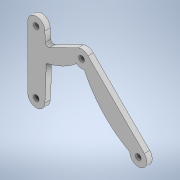
# Autodesk Inventor part: Bracket Concept MK5
Saved by Autodesk Inventor 2021 (Build 250183000, 183)
## iProperties
Created: 2021-05-11
Part Number: Bracket Concept MK5
Material: Generic
Document SubType Name: Modeling
Designer: Jawal
Density: 1 g/cm^3
Appearance: Default
Author: Jawal
Autodesk Inventor part; units mm, degrees
ref_plane "YZ Plane" through (0, 0, 0) normal (1, 0, 0) x (0, 1, 0)
ref_plane "XZ Plane" through (0, 0, 0) normal (0, 1, 0) x (-1, 0, 0)
ref_plane "XY Plane" through (0, 0, 0) normal (0, 0, 1) x (1, 0, 0)
sketch "Sketch1" plane through (0, 0, 0) normal (0, 0, 1) x (1, 0, 0)
  line L0 (-110, 70) -> (110, 70) construction
  line L1 (110, 70) -> (110, -70) construction
  line L2 (110, -70) -> (-110, -70) construction
  line L3 (-110, -70) -> (-110, 70) construction
  circle A0 centre (-90, 55) radius 5
  circle A1 centre (-90, -55) radius 5
  circle A2 centre (90, -55) radius 5
  circle A3 centre (-10, 45) radius 5
  line L4 (-67, 0) -> (-42, 0) construction
  line L5 (-42, 0) -> (-42, -30) construction
  line L6 (-42, -30) -> (-67, -30) construction
  line L7 (-67, -30) -> (-67, 0) construction
  circle A4 centre (-54.5, -11) radius 10 construction
  circle A5 centre (-63.5044, -24.4163) radius 3 construction
  circle A6 centre (-57.3559, -26.4695) radius 3 construction
  circle A7 centre (-51.263, -24.6531) radius 3 construction
  circle A8 centre (-45.3418, -26.5938) radius 3 construction
  arc A9 (-75, 55) -> (-105, 55) centre (-90, 55) ccw
  arc A10 (-105, -55) -> (-75, -55) centre (-90, -55) ccw
  arc A11 (75, -55) -> (100.6048, -44.3916) centre (90, -55) ccw
  line L8 (-105, 55) -> (-105, -55)
  line L9 (-66.6851, 34.062) -> (-16.5712, 58.484)
  arc A12 (-69.8902, 7.8152) -> (-19.1143, 33.0484) centre (-96.0046, 124.0681) ccw
  arc A13 (-75, -55) -> (-72.8183, 4.1339) centre (-763.2438, 0) ccw
  arc A14 (-73.8678, 38.2795) -> (-75, 55) centre (-763.2438, 0) ccw
  line L10 (1.1803, 55) -> (100.6048, -44.3916)
  arc A15 (-5.3208, 30.7166) -> (75, -55) centre (163.06, 108.0073) ccw
  arc A16 (-19.1143, 33.0484) -> (-5.3208, 30.7166) centre (-10, 45) ccw
  arc A17 (1.1803, 55) -> (-16.5712, 58.484) centre (-10, 45) ccw
  arc A18 (-73.8678, 38.2795) -> (-66.6851, 34.062) centre (-68.8755, 38.5567) ccw
  arc A19 (-69.8902, 7.8152) -> (-72.8183, 4.1339) centre (-69.0683, 4.1564) ccw
  point P0 (0, 0)
  dimension "d1" = 70
  dimension "d2" = 70
  dimension "d3" = 110
  dimension "d4" = 110
  dimension "d5" = 10
  dimension "d6" = 10
  dimension "d7" = 10
  dimension "d8" = 10
  dimension "d9" = 55
  dimension "d10" = 55
  dimension "d11" = 55
  dimension "d12" = 180
  dimension "d13" = 90
  dimension "d14" = 90
  dimension "d15" = 10
  dimension "d16" = 45
  dimension "d17" = 42
  dimension "d18" = 30
  dimension "d19" = 0
  dimension "d20" = 25
  dimension "d21" = 20
  dimension "d22" = 6
  dimension "d23" = 6
  dimension "d24" = 6
  dimension "d25" = 11
  dimension "d26" = 12.5
  dimension "d27" = 6
  dimension "d50" = 30
  dimension "d51" = 30
  dimension "d52" = 30
  dimension "d53" = 10
  dimension "d54" = 7.5
  constraints: 22 end point, 22 point on circle, 20 centre point, 6 tangent, 4 coincident, 4 parallel, 2 horizontal, 2 perpendicular, 1 vertical
  measures "d1" distance from line of point (0, 0) L2
  measures "d2" distance from line of point (0, 0) L0
  measures "d3" distance from line of L1 point (0, 0)
  measures "d4" distance from line of point (0, 0) L3
  measures "d5" diameter of A0
  measures "d6" diameter of A1
  measures "d7" diameter of A2
  measures "d8" diameter of A3
  measures "d9" vertical distance of point (0, 0) A0.centre
  measures "d10" vertical distance of point (0, 0) A1.centre
  measures "d11" vertical distance of A2.centre point (0, 0)
  measures "d12" distance of A2.centre A1.centre
  measures "d13" horizontal distance of point (0, 0) A0.centre
  measures "d14" horizontal distance of point (0, 0) A1.centre
  measures "d15" horizontal distance of point (0, 0) A3.centre
  measures "d16" vertical distance of point (0, 0) A3.centre
  measures "d17" distance from line of point (0, 0) L5
  measures "d18" distance of L4.end L5.end
  measures "d19" distance from line of L4 point (0, 0)
  measures "d20" distance of L5.end L6.end
  measures "d21" diameter of A4
  measures "d22" diameter of A5
  measures "d23" diameter of A6
  measures "d24" diameter of A7
  measures "d25" distance from line of L4 A4.centre
  measures "d26" distance from line of L7 A4.centre
  measures "d27" diameter of A8
  measures "d50" diameter of A9
  measures "d51" diameter of A10
  measures "d52" diameter of A11
  measures "d53" diameter of A18
  measures "d54" diameter of A19
extrude "Extrusion4" add sketch "Sketch1" along normal blind 9.4
equation "\"d1\" = d2"
equation "\"d4\" = d3"
equation "\"d10\" = d9"
equation "\"d11\" = d9"
equation "\"d14\" = d13"
equation "\"d26\" = 0.5 * d20"
body "Solid4"
